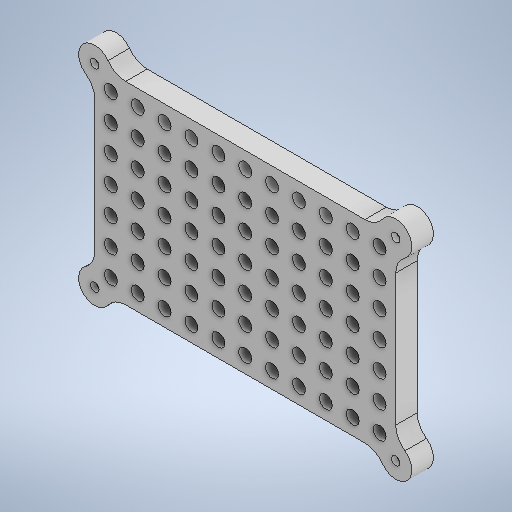
# Autodesk Inventor part: Top_Tip_Matrix
Saved by Autodesk Inventor 2025.1 (Build 291241000, 241)
## iProperties
Created: 2025-02-14
Part Number: Top_Tip_Matrix
Material: Generic
Document SubType Name: Modeling
Designer: m_kni
Density: 1 g/cm^3
Appearance: Default
Author: m_kni
## iProperties of the stored document Top_Tip_Matrix_3DPrint.ipt
Created: 2025-02-16
Part Number: Top_Tip_Matrix_3DPrint
Material: Generic
Document SubType Name: Modeling
Designer: m_kni
Density: 1 g/cm^3
Appearance: Default
Author: m_kni
Autodesk Inventor part; units mm, degrees
ref_plane "YZ Plane" through (0, 0, 0) normal (1, 0, 0) x (0, 1, 0)
ref_plane "XZ Plane" through (0, 0, 0) normal (0, 1, 0) x (-1, 0, 0)
ref_plane "XY Plane" through (0, 0, 0) normal (0, 0, 1) x (1, 0, 0)
sketch "Sketch1" plane through (0, 0, 0) normal (0, 0, 1) x (1, 0, 0)
  line L0 (55, -36) -> (-55, -36)
  line L1 (-55, -36) -> (-55, 36)
  line L2 (-55, 36) -> (55, 36)
  line L3 (55, -36) -> (-55, 36) construction
  line L4 (-55, -36) -> (55, 36) construction
  circle A0 centre (-49, 30) radius 2.425
  circle A1 centre (-49, 20) radius 2.425
  circle A2 centre (-49, 10) radius 2.425
  circle A3 centre (-49, 0) radius 2.425
  circle A4 centre (-49, -10) radius 2.425
  circle A5 centre (-49, -20) radius 2.425
  circle A6 centre (-49, -30) radius 2.425
  circle A7 centre (-39, 30) radius 2.425
  circle A8 centre (-39, 20) radius 2.425
  circle A9 centre (-39, 10) radius 2.425
  circle A10 centre (-39, 0) radius 2.425
  circle A11 centre (-39, -10) radius 2.425
  circle A12 centre (-39, -20) radius 2.425
  circle A13 centre (-39, -30) radius 2.425
  circle A14 centre (-29, 30) radius 2.425
  circle A15 centre (-29, 20) radius 2.425
  circle A16 centre (-29, 10) radius 2.425
  circle A17 centre (-29, 0) radius 2.425
  circle A18 centre (-29, -10) radius 2.425
  circle A19 centre (-29, -20) radius 2.425
  circle A20 centre (-29, -30) radius 2.425
  circle A21 centre (-19, 30) radius 2.425
  circle A22 centre (-19, 20) radius 2.425
  circle A23 centre (-19, 10) radius 2.425
  circle A24 centre (-19, 0) radius 2.425
  circle A25 centre (-19, -10) radius 2.425
  circle A26 centre (-19, -20) radius 2.425
  circle A27 centre (-19, -30) radius 2.425
  circle A28 centre (-9, 30) radius 2.425
  circle A29 centre (-9, 20) radius 2.425
  circle A30 centre (-9, 10) radius 2.425
  circle A31 centre (-9, 0) radius 2.425
  circle A32 centre (-9, -10) radius 2.425
  circle A33 centre (-9, -20) radius 2.425
  circle A34 centre (-9, -30) radius 2.425
  circle A35 centre (1, 30) radius 2.425
  circle A36 centre (1, 20) radius 2.425
  circle A37 centre (1, 10) radius 2.425
  circle A38 centre (1, 0) radius 2.425
  circle A39 centre (1, -10) radius 2.425
  circle A40 centre (1, -20) radius 2.425
  circle A41 centre (1, -30) radius 2.425
  circle A42 centre (11, 30) radius 2.425
  circle A43 centre (11, 20) radius 2.425
  circle A44 centre (11, 10) radius 2.425
  circle A45 centre (11, 0) radius 2.425
  circle A46 centre (11, -10) radius 2.425
  circle A47 centre (11, -20) radius 2.425
  circle A48 centre (11, -30) radius 2.425
  circle A49 centre (21, 30) radius 2.425
  circle A50 centre (21, 20) radius 2.425
  circle A51 centre (21, 10) radius 2.425
  circle A52 centre (21, 0) radius 2.425
  circle A53 centre (21, -10) radius 2.425
  circle A54 centre (21, -20) radius 2.425
  circle A55 centre (21, -30) radius 2.425
  circle A56 centre (31, 30) radius 2.425
  circle A57 centre (31, 20) radius 2.425
  circle A58 centre (31, 10) radius 2.425
  circle A59 centre (31, 0) radius 2.425
  circle A60 centre (31, -10) radius 2.425
  circle A61 centre (31, -20) radius 2.425
  circle A62 centre (31, -30) radius 2.425
  circle A63 centre (41, 30) radius 2.425
  circle A64 centre (41, 20) radius 2.425
  circle A65 centre (41, 10) radius 2.425
  circle A66 centre (41, 0) radius 2.425
  circle A67 centre (41, -10) radius 2.425
  circle A68 centre (41, -20) radius 2.425
  circle A69 centre (41, -30) radius 2.425
  circle A70 centre (51, 30) radius 2.425
  circle A71 centre (51, 20) radius 2.425
  circle A72 centre (51, 10) radius 2.425
  circle A73 centre (51, 0) radius 2.425
  circle A74 centre (51, -10) radius 2.425
  circle A75 centre (51, -20) radius 2.425
  circle A76 centre (51, -30) radius 2.425
  line L5 (-55, 36) -> (57, 36)
  line L6 (57, 36) -> (57, -36)
  line L7 (57, -36) -> (-55, -36)
  line L8 (-55, -36) -> (-55, 36)
  circle A77 centre (-55, 36) radius 6
  circle A78 centre (-55, -36) radius 6
  circle A79 centre (57, 36) radius 6
  circle A80 centre (57, -36) radius 6
  point P0 (0, 0)
  point P1 (57, 30)
  point P2 (-49, -36)
  point P3 (57, -30)
  point P4 (57, 30)
  point P5 (51, 36)
  point P6 (-49, 36)
  point P7 (-55, 30)
  point P8 (-55, -30)
  point P9 (-49, -36)
  point P10 (51, -36)
  dimension "d0" = 110
  dimension "d1" = 72
  dimension "d2" = 4.85
  dimension "d3" = 6
  dimension "d4" = 6
  dimension "d7" = 10
  dimension "d10" = 10
  dimension "d13" = 6
  dimension "d14" = 6
  dimension "d15" = 12
  dimension "d16" = 12
  dimension "d17" = 12
  dimension "d18" = 12
  constraints: 81 centre point, 18 end point, 5 coincident, 3 horizontal, 3 parallel, 2 midpoint, 2 perpendicular, 1 vertical, 152 other
  measures "d0" distance of L1.end L2.end
  measures "d1" distance of L0.end L1.end
  measures "d2" diameter of A0
  measures "d3" distance from line of A0.centre L2
  measures "d4" distance from line of A0.centre L1
  measures "d7" distance of A0.centre A1.centre
  measures "d10" distance of A0.centre A7.centre
  measures "d13" distance of point (57, 30) A70.centre
  measures "d14" distance of point (-49, -36) A6.centre
  measures "d15" diameter of A77
  measures "d16" diameter of A78
  measures "d17" diameter of A79
  measures "d18" diameter of A80
extrude "Extrusion1" add sketch "Sketch1" along normal blind 8
sketch "Sketch2" plane through (0, 0, 8) normal (0, 0, 1) x (1, 0, 0)
  arc A0 (-49, 36) -> (-55, 30) centre (-55, 36) ccw projected
  arc A1 (57, 30) -> (51, 36) centre (57, 36) ccw projected
  line L0 (51, 36) -> (-49, 36) projected
  arc A2 (-49, 36) -> (-55, 30) centre (-55, 36) ccw projected
  line L1 (-55, 30) -> (-55, -30) projected
  arc A3 (-55, -30) -> (-49, -36) centre (-55, -36) ccw projected
  line L2 (-49, -36) -> (51, -36) projected
  arc A4 (51, -36) -> (57, -30) centre (57, -36) ccw projected
  line L3 (57, -30) -> (57, 30) projected
  circle A5 centre (51, -10) radius 2.425 projected
  circle A6 centre (51, 10) radius 2.425 projected
  circle A7 centre (41, -30) radius 2.425 projected
  circle A8 centre (41, -10) radius 2.425 projected
  circle A9 centre (41, 10) radius 2.425 projected
  circle A10 centre (41, 30) radius 2.425 projected
  circle A11 centre (31, -20) radius 2.425 projected
  circle A12 centre (31, 0) radius 2.425 projected
  circle A13 centre (31, 20) radius 2.425 projected
  circle A14 centre (21, -30) radius 2.425 projected
  circle A15 centre (21, -10) radius 2.425 projected
  circle A16 centre (21, 10) radius 2.425 projected
  circle A17 centre (21, 30) radius 2.425 projected
  circle A18 centre (11, -20) radius 2.425 projected
  circle A19 centre (11, 0) radius 2.425 projected
  circle A20 centre (11, 20) radius 2.425 projected
  circle A21 centre (1, -30) radius 2.425 projected
  circle A22 centre (1, -10) radius 2.425 projected
  circle A23 centre (1, 10) radius 2.425 projected
  circle A24 centre (1, 30) radius 2.425 projected
  circle A25 centre (-9, -20) radius 2.425 projected
  circle A26 centre (-9, 0) radius 2.425 projected
  circle A27 centre (-9, 20) radius 2.425 projected
  circle A28 centre (-19, -30) radius 2.425 projected
  circle A29 centre (-19, -10) radius 2.425 projected
  circle A30 centre (-19, 10) radius 2.425 projected
  circle A31 centre (-19, 30) radius 2.425 projected
  circle A32 centre (-29, -20) radius 2.425 projected
  circle A33 centre (-29, 0) radius 2.425 projected
  circle A34 centre (-29, 20) radius 2.425 projected
  circle A35 centre (-39, -30) radius 2.425 projected
  circle A36 centre (-39, -10) radius 2.425 projected
  circle A37 centre (-39, 10) radius 2.425 projected
  circle A38 centre (-49, 20) radius 2.425 projected
  circle A39 centre (-49, 10) radius 2.425 projected
  circle A40 centre (-49, 0) radius 2.425 projected
  circle A41 centre (-49, -10) radius 2.425 projected
  circle A42 centre (-49, -20) radius 2.425 projected
  circle A43 centre (-39, 30) radius 2.425 projected
  circle A44 centre (-39, 20) radius 2.425 projected
  circle A45 centre (-39, 0) radius 2.425 projected
  circle A46 centre (-39, -20) radius 2.425 projected
  circle A47 centre (-29, 30) radius 2.425 projected
  circle A48 centre (-29, 10) radius 2.425 projected
  circle A49 centre (-29, -10) radius 2.425 projected
  circle A50 centre (-29, -30) radius 2.425 projected
  circle A51 centre (-19, 20) radius 2.425 projected
  circle A52 centre (-19, 0) radius 2.425 projected
  circle A53 centre (-19, -20) radius 2.425 projected
  circle A54 centre (-9, 30) radius 2.425 projected
  circle A55 centre (-9, 10) radius 2.425 projected
  circle A56 centre (-9, -10) radius 2.425 projected
  circle A57 centre (-9, -30) radius 2.425 projected
  circle A58 centre (1, 20) radius 2.425 projected
  circle A59 centre (1, 0) radius 2.425 projected
  circle A60 centre (1, -20) radius 2.425 projected
  circle A61 centre (11, 30) radius 2.425 projected
  circle A62 centre (11, 10) radius 2.425 projected
  circle A63 centre (11, -10) radius 2.425 projected
  circle A64 centre (11, -30) radius 2.425 projected
  circle A65 centre (21, 20) radius 2.425 projected
  circle A66 centre (21, 0) radius 2.425 projected
  circle A67 centre (21, -20) radius 2.425 projected
  circle A68 centre (31, 30) radius 2.425 projected
  circle A69 centre (31, 10) radius 2.425 projected
  circle A70 centre (31, -10) radius 2.425 projected
  circle A71 centre (31, -30) radius 2.425 projected
  circle A72 centre (41, 20) radius 2.425 projected
  circle A73 centre (41, 0) radius 2.425 projected
  circle A74 centre (41, -20) radius 2.425 projected
  circle A75 centre (51, 20) radius 2.425 projected
  circle A76 centre (51, 0) radius 2.425 projected
  circle A77 centre (51, -20) radius 2.425 projected
  circle A78 centre (51, -30) radius 2.425 projected
  circle A79 centre (51, 30) radius 2.425 projected
  circle A80 centre (-49, -30) radius 2.425 projected
  circle A81 centre (-49, 30) radius 2.425 projected
  circle A82 centre (-55, 36) radius 4
  circle A83 centre (-55, -36) radius 4
  circle A84 centre (57, -36) radius 4
  circle A85 centre (57, 36) radius 4
  point P0 (0, 0)
  dimension "d21" = 8
  dimension "d22" = 8
  dimension "d23" = 8
  dimension "d24" = 8
  constraints: 4 centre point, 4 coincident
  measures "d21" diameter of A82
  measures "d22" diameter of A83
  measures "d23" diameter of A84
  measures "d24" diameter of A85
extrude "Extrusion2" cut sketch "Sketch2" against normal blind 8 contours A82 | A83 | A84 | A85
sketch "Sketch3" plane through (0, 0, 8) normal (0, 0, 1) x (1, 0, 0)
  circle A0 centre (-55, 36) radius 4 projected
  circle A1 centre (-55, -36) radius 4 projected
  circle A2 centre (57, 36) radius 4 projected
  circle A3 centre (57, -36) radius 4 projected
  point P0 (0, 0)
extrude "Extrusion3" add sketch "Sketch3" against normal blind 2
sketch "Sketch4" plane through (0, 0, 8) normal (0, 0, 1) x (1, 0, 0)
  arc A0 (-49, 36) -> (-55, 30) centre (-55, 36) ccw projected
  arc A1 (57, 30) -> (51, 36) centre (57, 36) ccw projected
  arc A2 (-55, -30) -> (-49, -36) centre (-55, -36) ccw projected
  arc A3 (51, -36) -> (57, -30) centre (57, -36) ccw projected
  circle A4 centre (-55, 36) radius 1.6
  circle A5 centre (-55, -36) radius 4 projected
  circle A6 centre (-55, -36) radius 1.6
  circle A7 centre (57, 36) radius 1.6
  circle A8 centre (57, -36) radius 1.6
  point P0 (0, 0)
  dimension "d29" = 3.2
  dimension "d30" = 3.2
  dimension "d31" = 3.2
  dimension "d32" = 3.2
  constraints: 4 centre point, 4 coincident
  measures "d29" diameter of A4
  measures "d30" diameter of A6
  measures "d31" diameter of A7
  measures "d32" diameter of A8
extrude "Extrusion4" cut sketch "Sketch4" against normal blind 22.6375 contours A4 | A6 | A7 | A8
fillet "Fillet1" radius 8 8 edges at (-49, 36, 4) (51, 36, 4) (57, 30, 4) (57, -30, 4) (51, -36, 4) (-49, -36, 4) (-55, -30, 4) (-55, 30, 4)
body "Solid1"
